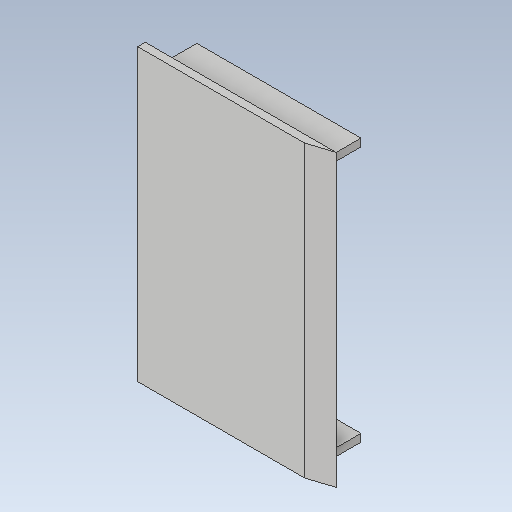
# Autodesk Inventor part: cover2
Saved by Autodesk Inventor 2020 (Build 240168000, 168)
## iProperties
Created: 2020-01-31
Part Number: cover2
Material: Ogólne
Document SubType Name: Modeling
Designer: blep
Density: 1 g/cm^3
Appearance: Domyślne
Author: blep
Autodesk Inventor part; units mm, degrees
ref_plane "YZ Plane" through (0, 0, 0) normal (1, 0, 0) x (0, 1, 0)
ref_plane "XZ Plane" through (0, 0, 0) normal (0, 1, 0) x (-1, 0, 0)
ref_plane "XY Plane" through (0, 0, 0) normal (0, 0, 1) x (1, 0, 0)
sketch "Sketch1" plane through (0, 0, 0) normal (0, 0, 1) x (1, 0, 0)
  line L0 (-22, 35) -> (22, 35) projected
  line L1 (22, 35) -> (22, -35) projected
  line L2 (22, -35) -> (-22, -35) projected
  line L3 (-25, -38) -> (25, -38) projected
  line L4 (25, -38) -> (25, 38) projected
  line L5 (25, 38) -> (-25, 38) projected
  line L6 (-25, 38) -> (-25, -38) projected
  line L7 (-22, -6.5359) -> (-22, 6.5359) projected
  arc A0 (-22, -6.5359) -> (-22, -13.4641) centre (-20, -10) ccw projected
  arc A1 (-22, 13.4641) -> (-22, 6.5359) centre (-20, 10) ccw projected
  line L8 (-22, 13.4641) -> (-22, 35) projected
  line L9 (-22, -35) -> (-22, -13.4641) projected
  point P0 (0, 0)
extrude "Extrusion1" add sketch "Sketch1" along normal blind 2 contours L0 L1 L2 L9 A0 L7 A1 L8 | L6 L5 L4 L3
sketch "Sketch2" plane through (-25, -38, 0) normal (0, -1, 0) x (1, 0, 0)
  line L0 (50, 0) -> (103.092, -17) construction
  line L1 (43.7539, 2) -> (50, 0)
  line L2 (0, 2) -> (50, 2) construction
  line L3 (50, 0) -> (50, 2) projected
  line L4 (43.7539, 2) -> (50, 2)
  line L5 (50, 2) -> (50, 0)
  point P0 (25, 0)
  constraints: 6 end point, 1 collinear, 1 horizontal, 1 perpendicular, 1 point on line
extrude "Extrusion2" cut sketch "Sketch2" against normal through all
sketch "Sketch3" plane through (0, 0, 0) normal (0, 0, -1) x (-1, 0, 0)
  line L0 (-22, -35) -> (22, -35) projected
  line L1 (22, 35) -> (-22, 35) projected
  line L2 (-22, 35) -> (-22, -35) projected
  line L3 (22, -35) -> (22, -13.4641) projected
  line L4 (22, 13.4641) -> (22, 35) projected
  line L5 (-21.5, -34.5) -> (21.5, -34.5)
  line L6 (21.5, -34.5) -> (21.5, -32.5)
  line L7 (21.5, -32.5) -> (-21.5, -32.5)
  line L8 (-21.5, -32.5) -> (-21.5, -34.5)
  line L9 (-21.5, 32.5) -> (21.5, 32.5)
  line L10 (21.5, 32.5) -> (21.5, 34.5)
  line L11 (21.5, 34.5) -> (-21.5, 34.5)
  line L12 (-21.5, 34.5) -> (-21.5, 32.5)
  point P0 (0, 0)
  dimension "d4" = 0.5
  dimension "d5" = 0.5
  dimension "d6" = 0.5
  dimension "d8" = 0.5
  dimension "d9" = 2
  dimension "d10" = 2
  constraints: 16 end point, 4 parallel, 2 horizontal, 2 perpendicular, 1 collinear, 1 point on line
  measures "d4" distance between parallel lines of L2 L8
  measures "d5" distance between parallel lines of L0 L5
  measures "d6" distance between parallel lines of L3 L6
  measures "d8" distance between parallel lines of L1 L11
  measures "d9" distance between parallel lines of L5 L7
  measures "d10" distance between parallel lines of L11 L9
extrude "Extrusion3" add sketch "Sketch3" along normal blind 10
equation "\"d5\" = d4"
equation "\"d6\" = d4"
equation "\"d8\" = d4"
equation "\"d10\" = d9"
body "Solid1"
